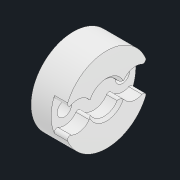
# Autodesk Inventor part: unit-base4
Saved by Autodesk Inventor 2021 (Build 250183000, 183)
## iProperties
Created: 2020-09-13
Part Number: unit-base4
Material: ABS プラスチック
Document SubType Name: Modeling
Designer: Yuta Kage
Mass: 0.883468 g
Surface Area: 8.24966 cm^2
Volume: 0.83346 cm^3
Density: 1.06 g/cm^3
Appearance: 滑らか - 白
Description: 3Dプリント
購入先: 印刷
在庫数: 0.0
Author: Yuta Kage
Autodesk Inventor part; units mm, degrees
ref_plane "YZ Plane" through (0, 0, 0) normal (1, 0, 0) x (0, 1, 0)
ref_plane "XZ Plane" through (0, 0, 0) normal (0, 1, 0) x (-1, 0, 0)
ref_plane "XY Plane" through (0, 0, 0) normal (0, 0, 1) x (1, 0, 0)
sketch "スケッチ1" plane through (0, 0, 0) normal (0, 0, 1) x (1, 0, 0)
  line L0 (0, 0) -> (0, 3.5)
  line L1 (0, 3.5) -> (0, 3.5)
  line L2 (0, 3.5) -> (0, 8)
  line L3 (0, 8) -> (6.3, 8)
  line L4 (6.3, 8) -> (6.3, 3)
  line L5 (6.3, 3) -> (3.8, 3)
  line L6 (3.8, 3) -> (3.8, 0)
  line L7 (3.8, 0) -> (0, 0)
  dimension "d0" = 3.5
  dimension "d1" = 3
  dimension "d2" = 2.5
  dimension "d4" = 0
  dimension "d5" = 8
  dimension "d34" = 3.8
  constraints: 16 end point, 7 perpendicular, 1 vertical
  measures "d0" distance of L0.start L0.end
  measures "d1" distance of L5.end L6.end
  measures "d2" distance of L4.end L5.end
  measures "d4" distance of L0.end L1.end
  measures "d5" distance from line of L0.start L3
  measures "d34" distance between parallel lines of L6 L2
revolve "回転1" add sketch "スケッチ1" angle 360 about axis through (3.8, 0, 0) along (-1, 0, 0)
sketch "スケッチ2" plane through (6.3, 0, 0) normal (1, 0, 0) x (0, 0, -1)
  point P0 (0, 0)
  point P1 (-5.5, 0)
  point P2 (5.5, 0)
  dimension "d10" = 5.5
  dimension "d11" = 5.5
  measures "d10" distance of point (0, 0) point (5.5, 0)
  measures "d11" distance of point (-5.5, 0) point (0, 0)
hole "穴1" at (6.3, 0, 5.5) at (6.3, 0, -5.5) direction (-1, 0, 0) diameter 2.7 end through all counterbore diameter 5.5 counterbore depth 2.5 clearance for "Socket Head Cap Screw" size "M2.5" standard "Ansi Metric M Profile"
chamfer "面取り5" distance 0.5 angle 45 2 edges at (6.3, -3, 0) (6.3, 3, 0)
fillet "フィレット2" radius 0.5 8 edges at (4.8, 0.8377, 2.8807) (4.8, 0.8377, -2.8807) (4.8, -0.8377, 2.8807) (4.8, -0.8377, -2.8807) (5.05, -1.3765, -7.8807) (5.05, 1.3765, -7.8807) (5.05, -1.3765, 7.8807) (5.05, 1.3765, 7.8807)
